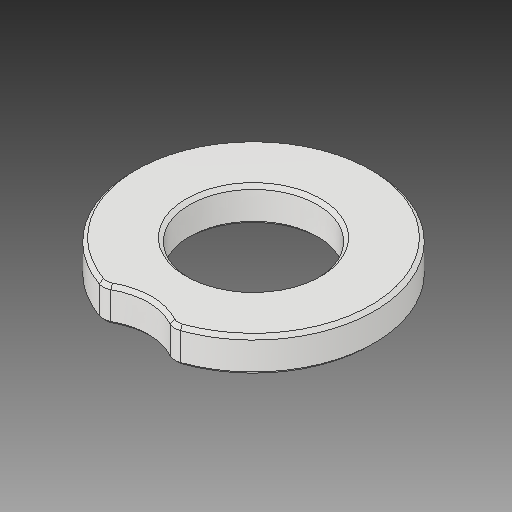
# Autodesk Inventor part: Motor Mount
Saved by Autodesk Inventor 2019.4 (Build 234330000, 330)
## iProperties
Created: 2019-03-01
Part Number: Motor Mount
Material: ABS Plastic
Document SubType Name: Modeling
Designer: Petar
Density: 1.06 g/cm^3
Appearance: Smooth - White
Mass: 3.54963 g
Surface Area: 20.9927 cm^2
Volume: 3.34871 cm^3
Author: Petar
Autodesk Inventor part; units mm, degrees
ref_plane "YZ Plane" through (0, 0, 0) normal (1, 0, 0) x (0, 1, 0)
ref_plane "XZ Plane" through (0, 0, 0) normal (0, 1, 0) x (-1, 0, 0)
ref_plane "XY Plane" through (0, 0, 0) normal (0, 0, 1) x (1, 0, 0)
sketch "Sketch1" plane through (0, 0, 0) normal (0, 1, 0) x (-1, 0, 0)
  circle A0 centre (0, 0) radius 9.25
  circle A1 centre (0, 0) radius 13.75 construction
  circle A2 centre (9.7227, -9.7227) radius 1.7
  line L0 (9.7227, -9.7227) -> (0, 0) construction
  circle A3 centre (9.7227, 9.7227) radius 1.7
  circle A4 centre (-9.7227, 9.7227) radius 1.7
  circle A5 centre (-9.7227, -9.7227) radius 1.7
  line L1 (0, 0) -> (0, -13.75) construction
  circle A6 centre (0, 0) radius 17.5
  circle A7 centre (0, 0) radius 10 construction
  line L2 (5, 16.7705) -> (0, 13.75) construction
  line L3 (0, 13.75) -> (-5, 16.7705) construction
  spline S0 degree 2 poles (5, 16.7705) (0, 13.75) (-5, 16.7705) knots 1 1 1 2 2 2
  line L4 (5, 16.7705) -> (-5, 16.7705) construction
  line L5 (0, 13.75) -> (0, 10) construction
  dimension "d10" = 20
  dimension "d0" = 18.5
  dimension "d2" = 3.4
  dimension "d6" = 360
  dimension "d8" = 45
  dimension "d11" = 10
  dimension "d30" = 7.5
  dimension "d31" = 3.75
  constraints: 8 end point, 7 centre point, 6 point on circle, 5 coincident, 2 vertical, 1 collinear, 1 horizontal, 1 vertical alignment, 15 other
  measures "d0" diameter of A0
  measures "d2" diameter of A2
  measures "d8" angle of L1 L0
  measures "d11" distance of L2.start L4.end
extrude "Extrusion1" add sketch "Sketch1" along normal blind 5 contours A2 | A3 | A4 | A5 | A6 S0 picked at (12.2147, -4.9313)
fillet "Fillet1" radius 2 2 edges at (-5, 2.5, 16.7705) (5, 2.5, 16.7705)
chamfer "Chamfer1" distance 0.5 angle 45 2 edges at (9.25, 5, 0) (9.25, 0, 0)
chamfer "Chamfer2" distance 0.5 angle 45 8 edges at (0, 5, -17.5) (-5.0769, 5, 16.5928) (0, 5, 15.2603) (5.0769, 5, 16.5928) (0, 0, -17.5) (-5.0769, 0, 16.5928) (0, 0, 15.2603) (5.0769, 0, 16.5928)
body "Solid1"
